Autodesk Inventor part; units mm, degrees
(part 2 of 2)
extrude "Extrusion24" cut sketch "Sketch28" against normal blind 1 contours L33 L34 L10 L12 | L12 L10 S18 L36 L29 L30 L31 L32 L33 | L12 L35 S16 S17 S18 L10 | L10 L34 L35 L12 | S2 S3 S4 S5 L13 L14 S6 S7 S8 S9 L10 | L10 S9 S10 S11 S12 S13 L15 L16 S14 S15 S0 S1 S2 | L26 L27 L28 L17 L18 L19 L20 L10 | L10 L20 L21 L22 L23 L24 L25 L26 | S25 S26 S27 S28 L40 L41 S29 S30 S31 S32 L10 | L10 S32 S33 S34 S35 S36 L42 L43 S37 S38 S23 S24 S25 bodies 3
chamfer "Chamfer2" distance 0.5 angle 45 69 edges at (3.5434, 22.1781, 13.5) (1.331, 22.8406, 13.5) (-2.8323, 22.4212, 13.5) (-6.3513, 18.4524, 13.5) (-6.3391, 11.8155, 13.5) (-2.814, 7.9075, 13.5) (1.3371, 7.5246, 13.5) (3.6102, 8.26, 13.5) (4.5462, 9.8949, 13.5) (3.7622, 10.527, 13.5) (4.4733, 11.0861, 13.5) (3.7075, 19.8625, 13.5) (1.4526, 21.0476, 13.5) (-1.9145, 20.8532, 13.5) (-4.4003, 17.7778, 13.5) (-4.3821, 12.5144, 13.5) (-1.8902, 9.5181, 13.5) (1.5012, 9.354, 13.5) (4.4672, 19.279, 13.5) (4.5462, 20.4824, 13.5) (5.8225, 21.9168, 13.5) (8.7277, 22.6826, 13.5) (6.7767, 21.151, 13.5) (7.731, 15.1826, 13.5) (9.7245, 15.1826, 13.5) (10.6787, 21.151, 13.5) (11.6329, 21.9168, 13.5) (8.7277, 7.6826, 13.5) (11.6329, 8.4484, 13.5) (10.6787, 9.2142, 13.5) (6.7767, 9.2142, 13.5) (5.8225, 8.4484, 13.5) (14.1005, 15.1826, 13.5) (16.0332, 22.6826, 13.5) (20.1236, 22.5428, 13.5) (23.0288, 20.5857, 13.5) (22.6459, 15.8572, 13.5) (16.9692, 15.3163, 13.5) (19.3942, 15.4682, 13.5) (16.094, 18.1364, 13.5) (19.4672, 20.841, 13.5) (17.0847, 20.9565, 13.5) (21.175, 19.6133, 13.5) (21.1994, 17.091, 13.5) (17.2366, 13.651, 13.5) (20.7496, 10.6668, 13.5) (16.094, 10.6668, 13.5) (15.0972, 7.6826, 13.5) (23.0409, 10.9464, 13.5) (24.4145, 7.6826, 13.5) (26.5417, 11.8155, 13.5) (26.5296, 18.4524, 13.5) (28.4988, 12.5144, 13.5) (28.4806, 17.7778, 13.5) (30.0669, 7.9075, 13.5) (34.218, 7.5246, 13.5) (30.9907, 9.5181, 13.5) (34.3821, 9.354, 13.5) (30.0486, 22.4212, 13.5) (34.2119, 22.8406, 13.5) (30.9664, 20.8532, 13.5) (34.3335, 21.0476, 13.5) (36.5883, 19.8625, 13.5) (37.4271, 20.4824, 13.5) (36.4242, 22.1781, 13.5) (37.4271, 9.8949, 13.5) (36.643, 10.527, 13.5) (36.4911, 8.26, 13.5) (37.3541, 11.0861, 13.5)
ref_plane "Work Plane8" through (15, 0, 0) normal (1, 0, 0) x (0, 0, -1)
ref_plane "Work Plane11" through (15, 30.4, 0) normal (-1, 0, 0) x (0, 0, -1)
ref_plane "Work Plane12" through (15, 30.4, 0) normal (-1, 0, 0) x (0, 0, -1)
equation "\"d4\" = d0"
body "Solid1"
